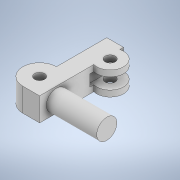
# Autodesk Inventor part: stuur_ARMPJE
Saved by Autodesk Inventor 2022 (Build 260153000, 153)
## iProperties
Created: 2021-11-25
Part Number: stuur_ARMPJE
Material: Generic
Document SubType Name: Modeling
Designer: keemi
Density: 1 g/cm^3
Appearance: Default
Author: keemi
Autodesk Inventor part; units mm, degrees
ref_plane "YZ Plane" through (0, 0, 0) normal (1, 0, 0) x (0, 1, 0)
ref_plane "XZ Plane" through (0, 0, 0) normal (0, 1, 0) x (-1, 0, 0)
ref_plane "XY Plane" through (0, 0, 0) normal (0, 0, 1) x (1, 0, 0)
sketch "Sketch1" plane through (0, 0, 0) normal (0, 1, 0) x (-1, 0, 0)
  circle A0 centre (0, 0) radius 1.5
  circle A1 centre (0, 0) radius 5
  line L0 (-5, 0) -> (-5, 5)
  line L1 (-5, 5) -> (0, 5)
  line L2 (-5, 0) -> (-5, -20)
  line L3 (-5, -20) -> (-1.5, -20)
  line L4 (-5, -20) -> (0, -20)
  line L5 (0, -20) -> (0, -5)
  dimension "d0" = 3
  dimension "d1" = 10
  dimension "d2" = 20
  constraints: 12 end point, 3 point on circle, 2 centre point, 2 coincident, 2 perpendicular, 2 point on line, 2 tangent, 1 vertical
  measures "d0" diameter of A0
  measures "d1" diameter of A1
  measures "d2" distance of L0.start L2.end
extrude "Extrusion1" add sketch "Sketch1" along normal blind 7
sketch "Sketch2" plane through (5, 0, 5) normal (1, 0, 0) x (0, 0, -1)
  line L0 (10, 7) -> (0, 7) projected
  line L1 (0, 7) -> (0, 3.5)
  line L2 (0, 0) -> (25, 0) projected
  line L3 (0, 3.5) -> (5, 3.5)
  circle A0 centre (5, 3.5) radius 3
  point P0 (5, 0)
  dimension "d5" = 3.5
  dimension "d6" = 6
  constraints: 4 end point, 2 perpendicular, 1 centre point, 1 coincident
  measures "d5" distance of L0.end L1.end
  measures "d6" diameter of A0
extrude "Extrusion2" add sketch "Sketch2" along normal blind 15
sketch "Sketch3" plane through (5, 0, 5) normal (1, 0, 0) x (0, 0, -1)
  point P0 (5, 0)
sketch "Sketch4" plane through (0, 7, 0) normal (0, 1, 0) x (1, 0, 0)
  line L0 (5, -5) -> (5, 20) projected
  line L1 (5, 20) -> (5, 15)
  line L2 (5, 20) -> (5, 17)
  line L3 (5, 15) -> (6, 15)
  circle A0 centre (6, 15) radius 1.5
  circle A1 centre (6, 15) radius 4
  point P0 (0, 0)
  dimension "d10" = 3
  dimension "d11" = 1
  dimension "d12" = 3
  dimension "d13" = 8
  constraints: 6 end point, 2 centre point, 2 coincident, 2 point on line, 1 perpendicular
  measures "d10" distance of L0.end L2.end
  measures "d11" distance of L1.end L3.end
  measures "d12" diameter of A0
  measures "d13" diameter of A1
extrude "Extrusion3" add sketch "Sketch4" against normal blind 7 contours A1 L0 A0 | L0 A0 A1
sketch "Sketch5" plane through (0, 7, 0) normal (0, 1, 0) x (1, 0, 0)
  arc A0 (5, 13.882) -> (5, 16.118) centre (6, 15) ccw projected
  circle A1 centre (6, 15) radius 1.5
  point P0 (0, 0)
  point P1 (5, 13.882)
  constraints: 1 centre point, 1 coincident
extrude "Extrusion4" cut sketch "Sketch5" against normal blind 7
sketch "Sketch6" plane through (5, 0, -20) normal (1, 0, 0) x (0, 0, -1)
  line L0 (0, 7) -> (-15, 7) projected
  line L1 (0, 7) -> (0, 3.5)
  line L2 (0, 0) -> (0, 7) projected
  line L3 (0, 3.5) -> (0, 5.2)
  line L4 (0, 5.2) -> (-10, 5.2)
  line L5 (-10, 5.2) -> (-10, 1.8)
  line L6 (-10, 1.8) -> (0, 1.8)
  line L7 (0, 1.8) -> (0, 5.2)
  point P0 (-20, 0)
  point P1 (0, 1.8)
  point P2 (0, 5.2)
  dimension "d18" = 1.7
  dimension "d19" = 10
  dimension "d20" = 3.4
  constraints: 12 end point, 2 parallel, 1 horizontal, 1 midpoint, 1 perpendicular, 1 point on line
  measures "d18" distance of L1.end L3.end
  measures "d19" distance of L6.end L5.end
  measures "d20" distance of L5.end L4.end
extrude "Extrusion5" cut sketch "Sketch6" along normal blind 7 and the other way blind 1
body "Solid1"
